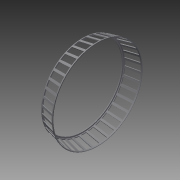
# Autodesk Inventor part: 32913_cage
Saved by Autodesk Inventor 2014 SP2 (Build 180246200, 246)
## iProperties
Created: 2018-11-17
Part Number: 32913_cage
Material: Generic
Catalog Web Link: www.cadenas.de
Description: BT1_001_101_cage-Tapered roller bearings, single row
Vendor: SKF
Document SubType Name: Modeling
Designer: psadmin
Manufacturer: SKF
Mass: 1.11318 g
Surface Area: 45.7917 cm^2
Volume: 1.11318 cm^3
Density: 1 g/cm^3
Appearance: PSOLRGB-175-175-175
Category: PARTsolutions
Company: SKF
Title: 32913_cage
Author: Cadenas PARTsolutions
Comments: Tapered roller bearings, single row
PSOL_IDENT_0: {$CADENAS_DATA\23d-libs\skf\bearings_units_and_housings\roller_bearings\tapered_roller_bearings\tape
PSOL_IDENT_1: red_roller_bearings_single_row\parts\bt1_001_101_cage.prj},172 {VTYP=3D},{NB=32913_cage},{LINA=32913
PSOL_IDENT_2: _cage},{NN=BT1_001_101_cage},{DATE=14.08.2018 07:35:10},{GEOMDATE=27.06.2018 08:15:48},{VERSION=},{L
PSOL_IDENT_3: INEID=3110},{WBVAR=},{WBNUMERIC=}  {NB=32913_cage},{LINA=32913_cage},{KT=DUMMY},{DESIGNATION=32913},
PSOL_IDENT_4: {DD=65.000},{D=90.000},{T=17.000},{DD1=78.8000},{D1=MIN},{B=17.000},{C=14.000},{C1=MIN},{R12=1.0},{R
PSOL_IDENT_5: 34=1.0},{AA=16.53733},{PITCH=77.207},{DW=5.200},{LW=12.200},{RANGLE=1.600},{ALPHA=13.250},{DDAMAX=71
PSOL_IDENT_6: },{DDAMIN=73.0},{DAMIN=83},{DAMAX=83.0},{DBMIN=86},{CA=3},{CB=3.0},{RA=1.0},{RB=1.0},{LOAD1=54.700},
PSOL_IDENT_7: {LOAD2=80.000},{LOAD3=8.150},{SPEED1=5600},{SPEED2=6700},{EE=0.35},{Y=1.70},{Y0=0.9},{Y1=0},{X1=1},{
PSOL_IDENT_8: X2=0.4},{X0=0.5},{Z=36},{II=1},{R1=0.00000231},{R2=10.9},{S1=0.009},{S2=2},{KZ=6},{KL=0.7},{BF=2},{M
PSOL_IDENT_9: ASS=0.323},{PIM=PIM_BT1_001},{DESIGN=trb1},{HELP=0.000}
NN: BT1_001_101_cage
NT: Tapered roller bearings, single row
NB: 32913_cage
NBSYN: $DESIGNATION._cage
LINA: 32913_cage
DESIGNATION: 32913
DD: 65
D: 90
T: 17
DD1: 78.8
D1: 0
B: 17
C: 14
C1: 0
R12: 1
R34: 1
AA: 16.53733
PITCH: 77.207
DW: 5.2
LW: 12.2
RANGLE: 1.6
ALPHA: 13.25
DDAMAX: 71
DDAMIN: 73
DAMIN: 83
DAMAX: 83
DBMIN: 86
CA: 3
CB: 3
RA: 1
RB: 1
LOAD1: 54.7
LOAD2: 80
LOAD3: 8.15
SPEED1: 5600
SPEED2: 6700
EE: 0.35
Y: 1.7
Y0: 0.9
Y1: 0
X1: 1
X2: 0.4
X0: 0.5
Z: 36
II: 1
R1: 0.00000231
R2: 10.9
S1: 0.009
S2: 2
KZ: 6
KL: 0.7
BF: 2
MASS: 0.323
PIM: PIM_BT1_001
SUPPLIER: SKF
ARTICLENO: 32913_cage
BOMINFO: 32913_cage
CREATOR: CADENAS GmbH
Autodesk Inventor part; units mm, degrees
ref_plane "YZ Plane" through (0, 0, 0) normal (1, 0, 0) x (0, 1, 0)
ref_plane "XZ Plane" through (0, 0, 0) normal (0, 1, 0) x (-1, 0, 0)
ref_plane "XY Plane" through (0, 0, 0) normal (0, 0, 1) x (1, 0, 0)
sketch "Sketch_1" plane through (0, 0, 0) normal (0, 0, 1) x (1, 0, 0)
  line L0 (0.4725, 0) -> (-0.1775, 0)
  line L1 (-0.1775, 38.1882) -> (-0.1775, 36.9611)
  line L2 (-0.1775, 36.9611) -> (0.4725, 36.9611)
  line L3 (0.4725, 36.9611) -> (0.4725, 38.1882)
  line L4 (0.4725, 38.1882) -> (14.3525, 41.565)
  line L5 (14.3525, 41.565) -> (14.2035, 42.1977)
  line L6 (14.2035, 42.1977) -> (0.3189, 38.8198)
  arc A0 (0.3189, 38.8198) -> (-0.1775, 38.1882) centre (0.4725, 38.1882) ccw
  constraints: 14 end point, 2 point on circle, 1 centre point
revolve "Revolution1" add sketch "Sketch_1" angle 360 about axis through (0.4725, 0, 0) along (1, 0, 0)
sketch "Sketch_2" plane through (7.1413, 0, 0) normal (1, 0, 0) x (0, 0, -1)
  line L0 (-43.8035, -2.7696) -> (-19.2633, -1.218)
  arc A0 (-19.2633, -1.218) -> (-19.1821, -2.1456) centre (0, 0) ccw
  line L1 (-19.1821, -2.1456) -> (-43.619, -4.8789)
  line L2 (-43.619, -4.8789) -> (-42.6571, -10.3339)
  line L3 (-42.6571, -10.3339) -> (-18.7591, -4.5445)
  arc A1 (-18.7591, -4.5445) -> (-18.5181, -5.4439) centre (0, 0) ccw
  line L4 (-18.5181, -5.4439) -> (-42.1091, -12.3791)
  line L5 (-42.1091, -12.3791) -> (-40.2146, -17.5842)
  line L6 (-40.2146, -17.5842) -> (-17.685, -7.7329)
  arc A2 (-17.685, -7.7329) -> (-17.2915, -8.5769) centre (0, 0) ccw
  line L7 (-17.2915, -8.5769) -> (-39.3197, -19.5032)
  line L8 (-39.3197, -19.5032) -> (-36.5502, -24.3003)
  line L9 (-36.5502, -24.3003) -> (-16.0735, -10.6864)
  arc A3 (-16.0735, -10.6864) -> (-15.5394, -11.4492) centre (0, 0) ccw
  line L10 (-15.5394, -11.4492) -> (-35.3357, -26.0347)
  line L11 (-35.3357, -26.0347) -> (-31.7752, -30.278)
  line L12 (-31.7752, -30.278) -> (-13.9736, -13.3152)
  arc A4 (-13.9736, -13.3152) -> (-13.3152, -13.9736) centre (0, 0) ccw
  line L13 (-13.3152, -13.9736) -> (-30.278, -31.7752)
  line L14 (-30.278, -31.7752) -> (-26.0347, -35.3357)
  line L15 (-26.0347, -35.3357) -> (-11.4492, -15.5394)
  arc A5 (-11.4492, -15.5394) -> (-10.6864, -16.0735) centre (0, 0) ccw
  line L16 (-10.6864, -16.0735) -> (-24.3003, -36.5502)
  line L17 (-24.3003, -36.5502) -> (-19.5032, -39.3197)
  line L18 (-19.5032, -39.3197) -> (-8.5769, -17.2915)
  arc A6 (-8.5769, -17.2915) -> (-7.7329, -17.685) centre (0, 0) ccw
  line L19 (-7.7329, -17.685) -> (-17.5842, -40.2146)
  line L20 (-17.5842, -40.2146) -> (-12.3791, -42.1091)
  line L21 (-12.3791, -42.1091) -> (-5.4439, -18.5181)
  arc A7 (-5.4439, -18.5181) -> (-4.5445, -18.7591) centre (0, 0) ccw
  line L22 (-4.5445, -18.7591) -> (-10.3339, -42.6571)
  line L23 (-10.3339, -42.6571) -> (-4.8789, -43.619)
  line L24 (-4.8789, -43.619) -> (-2.1456, -19.1821)
  arc A8 (-2.1456, -19.1821) -> (-1.218, -19.2633) centre (0, 0) ccw
  line L25 (-1.218, -19.2633) -> (-2.7696, -43.8035)
  line L26 (-2.7696, -43.8035) -> (2.7696, -43.8035)
  line L27 (2.7696, -43.8035) -> (1.218, -19.2633)
  arc A9 (1.218, -19.2633) -> (2.1456, -19.1821) centre (0, 0) ccw
  line L28 (2.1456, -19.1821) -> (4.8789, -43.619)
  line L29 (4.8789, -43.619) -> (10.3339, -42.6571)
  line L30 (10.3339, -42.6571) -> (4.5445, -18.7591)
  arc A10 (4.5445, -18.7591) -> (5.4439, -18.5181) centre (0, 0) ccw
  line L31 (5.4439, -18.5181) -> (12.3791, -42.1091)
  line L32 (12.3791, -42.1091) -> (17.5842, -40.2146)
  line L33 (17.5842, -40.2146) -> (7.7329, -17.685)
  arc A11 (7.7329, -17.685) -> (8.5769, -17.2915) centre (0, 0) ccw
  line L34 (8.5769, -17.2915) -> (19.5032, -39.3197)
  line L35 (19.5032, -39.3197) -> (24.3003, -36.5502)
  line L36 (24.3003, -36.5502) -> (10.6864, -16.0735)
  arc A12 (10.6864, -16.0735) -> (11.4492, -15.5394) centre (0, 0) ccw
  line L37 (11.4492, -15.5394) -> (26.0347, -35.3357)
  line L38 (26.0347, -35.3357) -> (30.278, -31.7752)
  line L39 (30.278, -31.7752) -> (13.3152, -13.9736)
  arc A13 (13.3152, -13.9736) -> (13.9736, -13.3152) centre (0, 0) ccw
  line L40 (13.9736, -13.3152) -> (31.7752, -30.278)
  line L41 (31.7752, -30.278) -> (35.3357, -26.0347)
  line L42 (35.3357, -26.0347) -> (15.5394, -11.4492)
  arc A14 (15.5394, -11.4492) -> (16.0735, -10.6864) centre (0, 0) ccw
  line L43 (16.0735, -10.6864) -> (36.5502, -24.3003)
  line L44 (36.5502, -24.3003) -> (39.3197, -19.5032)
  line L45 (39.3197, -19.5032) -> (17.2915, -8.5769)
  arc A15 (17.2915, -8.5769) -> (17.685, -7.7329) centre (0, 0) ccw
  line L46 (17.685, -7.7329) -> (40.2146, -17.5842)
  line L47 (40.2146, -17.5842) -> (42.1091, -12.3791)
  line L48 (42.1091, -12.3791) -> (18.5181, -5.4439)
  arc A16 (18.5181, -5.4439) -> (18.7591, -4.5445) centre (0, 0) ccw
  line L49 (18.7591, -4.5445) -> (42.6571, -10.3339)
  line L50 (42.6571, -10.3339) -> (43.619, -4.8789)
  line L51 (43.619, -4.8789) -> (19.1821, -2.1456)
  arc A17 (19.1821, -2.1456) -> (19.2633, -1.218) centre (0, 0) ccw
  line L52 (19.2633, -1.218) -> (43.8035, -2.7696)
  line L53 (43.8035, -2.7696) -> (43.8035, 2.7696)
  line L54 (43.8035, 2.7696) -> (19.2633, 1.218)
  arc A18 (19.2633, 1.218) -> (19.1821, 2.1456) centre (0, 0) ccw
  line L55 (19.1821, 2.1456) -> (43.619, 4.8789)
  line L56 (43.619, 4.8789) -> (42.6571, 10.3339)
  line L57 (42.6571, 10.3339) -> (18.7591, 4.5445)
  arc A19 (18.7591, 4.5445) -> (18.5181, 5.4439) centre (0, 0) ccw
  line L58 (18.5181, 5.4439) -> (42.1091, 12.3791)
  line L59 (42.1091, 12.3791) -> (40.2146, 17.5842)
  line L60 (40.2146, 17.5842) -> (17.685, 7.7329)
  arc A20 (17.685, 7.7329) -> (17.2915, 8.5769) centre (0, 0) ccw
  line L61 (17.2915, 8.5769) -> (39.3197, 19.5032)
  line L62 (39.3197, 19.5032) -> (36.5502, 24.3003)
  line L63 (36.5502, 24.3003) -> (16.0735, 10.6864)
  arc A21 (16.0735, 10.6864) -> (15.5394, 11.4492) centre (0, 0) ccw
  line L64 (15.5394, 11.4492) -> (35.3357, 26.0347)
  line L65 (35.3357, 26.0347) -> (31.7752, 30.278)
  line L66 (31.7752, 30.278) -> (13.9736, 13.3152)
  arc A22 (13.9736, 13.3152) -> (13.3152, 13.9736) centre (0, 0) ccw
  line L67 (13.3152, 13.9736) -> (30.278, 31.7752)
  line L68 (30.278, 31.7752) -> (26.0347, 35.3357)
  line L69 (26.0347, 35.3357) -> (11.4492, 15.5394)
  arc A23 (11.4492, 15.5394) -> (10.6864, 16.0735) centre (0, 0) ccw
  line L70 (10.6864, 16.0735) -> (24.3003, 36.5502)
  line L71 (24.3003, 36.5502) -> (19.5032, 39.3197)
  line L72 (19.5032, 39.3197) -> (8.5769, 17.2915)
  arc A24 (8.5769, 17.2915) -> (7.7329, 17.685) centre (0, 0) ccw
  line L73 (7.7329, 17.685) -> (17.5842, 40.2146)
  line L74 (17.5842, 40.2146) -> (12.3791, 42.1091)
  line L75 (12.3791, 42.1091) -> (5.4439, 18.5181)
  arc A25 (5.4439, 18.5181) -> (4.5445, 18.7591) centre (0, 0) ccw
  line L76 (4.5445, 18.7591) -> (10.3339, 42.6571)
  line L77 (10.3339, 42.6571) -> (4.8789, 43.619)
  line L78 (4.8789, 43.619) -> (2.1456, 19.1821)
  arc A26 (2.1456, 19.1821) -> (1.218, 19.2633) centre (0, 0) ccw
  line L79 (1.218, 19.2633) -> (2.7696, 43.8035)
  line L80 (2.7696, 43.8035) -> (-2.7696, 43.8035)
  line L81 (-2.7696, 43.8035) -> (-1.218, 19.2633)
  arc A27 (-1.218, 19.2633) -> (-2.1456, 19.1821) centre (0, 0) ccw
  line L82 (-2.1456, 19.1821) -> (-4.8789, 43.619)
  line L83 (-4.8789, 43.619) -> (-10.3339, 42.6571)
  line L84 (-10.3339, 42.6571) -> (-4.5445, 18.7591)
  arc A28 (-4.5445, 18.7591) -> (-5.4439, 18.5181) centre (0, 0) ccw
  line L85 (-5.4439, 18.5181) -> (-12.3791, 42.1091)
  line L86 (-12.3791, 42.1091) -> (-17.5842, 40.2146)
  line L87 (-17.5842, 40.2146) -> (-7.7329, 17.685)
  arc A29 (-7.7329, 17.685) -> (-8.5769, 17.2915) centre (0, 0) ccw
  line L88 (-8.5769, 17.2915) -> (-19.5032, 39.3197)
  line L89 (-19.5032, 39.3197) -> (-24.3003, 36.5502)
  line L90 (-24.3003, 36.5502) -> (-10.6864, 16.0735)
  arc A30 (-10.6864, 16.0735) -> (-11.4492, 15.5394) centre (0, 0) ccw
  line L91 (-11.4492, 15.5394) -> (-26.0347, 35.3357)
  line L92 (-26.0347, 35.3357) -> (-30.278, 31.7752)
  line L93 (-30.278, 31.7752) -> (-13.3152, 13.9736)
  arc A31 (-13.3152, 13.9736) -> (-13.9736, 13.3152) centre (0, 0) ccw
  line L94 (-13.9736, 13.3152) -> (-31.7752, 30.278)
  line L95 (-31.7752, 30.278) -> (-35.3357, 26.0347)
  line L96 (-35.3357, 26.0347) -> (-15.5394, 11.4492)
  arc A32 (-15.5394, 11.4492) -> (-16.0735, 10.6864) centre (0, 0) ccw
  line L97 (-16.0735, 10.6864) -> (-36.5502, 24.3003)
  line L98 (-36.5502, 24.3003) -> (-39.3197, 19.5032)
  line L99 (-39.3197, 19.5032) -> (-17.2915, 8.5769)
  arc A33 (-17.2915, 8.5769) -> (-17.685, 7.7329) centre (0, 0) ccw
  line L100 (-17.685, 7.7329) -> (-40.2146, 17.5842)
  line L101 (-40.2146, 17.5842) -> (-42.1091, 12.3791)
  line L102 (-42.1091, 12.3791) -> (-18.5181, 5.4439)
  arc A34 (-18.5181, 5.4439) -> (-18.7591, 4.5445) centre (0, 0) ccw
  line L103 (-18.7591, 4.5445) -> (-42.6571, 10.3339)
  line L104 (-42.6571, 10.3339) -> (-43.619, 4.8789)
  line L105 (-43.619, 4.8789) -> (-19.1821, 2.1456)
  arc A35 (-19.1821, 2.1456) -> (-19.2633, 1.218) centre (0, 0) ccw
  line L106 (-19.2633, 1.218) -> (-43.8035, 2.7696)
  line L107 (-43.8035, 2.7696) -> (-43.8035, -2.7696)
  constraints: 216 end point, 72 point on circle, 36 centre point
extrude "Extrusion1" cut sketch "Sketch_2" along normal mid plane 12.19
ref_plane "cage_XY" through (0, 0, 0) normal (0, 0, 1) x (1, 0, 0)
ref_plane "cage_YZ" through (0, 0, 0) normal (1, 0, 0) x (0, 1, 0)
ref_plane "cage_ZX" through (0, 0, 0) normal (0, 1, 0) x (0, 0, 1)
ref_plane "roller1_XY" through (0, 38.6035, 0) normal (1, 0, 0) x (0, 0, -1)
ref_plane "roller1_YZ" through (0, 38.6035, 0) normal (0, 0, -1) x (0, 1, 0)
ref_plane "roller1_ZX" through (0, 38.6035, 0) normal (0, 1, 0) x (1, 0, 0)
ref_plane "roller10_XY" through (0, 0, 38.6035) normal (1, 0, 0) x (0, 1, 0)
ref_plane "roller10_YZ" through (0, 0, 38.6035) normal (0, 1, 0) x (0, 0, 1)
ref_plane "roller10_ZX" through (0, 0, 38.6035) normal (0, 0, 1) x (1, 0, 0)
ref_plane "roller11_XY" through (0, -6.7034, 38.017) normal (1, 0, 0) x (0, 0.9848078, 0.1736482)
ref_plane "roller11_YZ" through (0, -6.7034, 38.017) normal (0, 0.9848078, 0.1736482) x (0, -0.1736482, 0.9848078)
ref_plane "roller11_ZX" through (0, -6.7034, 38.017) normal (0, -0.1736482, 0.9848078) x (1, 0, 0)
ref_plane "roller12_XY" through (0, -13.2032, 36.2754) normal (1, 0, 0) x (0, 0.9396926, 0.3420201)
ref_plane "roller12_YZ" through (0, -13.2032, 36.2754) normal (0, 0.9396926, 0.3420201) x (0, -0.3420201, 0.9396926)
ref_plane "roller12_ZX" through (0, -13.2032, 36.2754) normal (0, -0.3420201, 0.9396926) x (1, 0, 0)
ref_plane "roller13_XY" through (0, -19.3017, 33.4316) normal (1, 0, 0) x (0, 0.8660254, 0.5)
ref_plane "roller13_YZ" through (0, -19.3017, 33.4316) normal (0, 0.8660254, 0.5) x (0, -0.5, 0.8660254)
ref_plane "roller13_ZX" through (0, -19.3017, 33.4316) normal (0, -0.5, 0.8660254) x (1, 0, 0)
ref_plane "roller14_XY" through (0, -24.8139, 29.572) normal (1, 0, 0) x (0, 0.7660444, 0.6427876)
ref_plane "roller14_YZ" through (0, -24.8139, 29.572) normal (0, 0.7660444, 0.6427876) x (0, -0.6427876, 0.7660444)
ref_plane "roller14_ZX" through (0, -24.8139, 29.572) normal (0, -0.6427876, 0.7660444) x (1, 0, 0)
ref_plane "roller15_XY" through (0, -29.572, 24.8139) normal (1, 0, 0) x (0, 0.6427876, 0.7660444)
ref_plane "roller15_YZ" through (0, -29.572, 24.8139) normal (0, 0.6427876, 0.7660444) x (0, -0.7660444, 0.6427876)
ref_plane "roller15_ZX" through (0, -29.572, 24.8139) normal (0, -0.7660444, 0.6427876) x (1, 0, 0)
ref_plane "roller16_XY" through (0, -33.4316, 19.3017) normal (1, 0, 0) x (0, 0.5, 0.8660254)
ref_plane "roller16_YZ" through (0, -33.4316, 19.3017) normal (0, 0.5, 0.8660254) x (0, -0.8660254, 0.5)
ref_plane "roller16_ZX" through (0, -33.4316, 19.3017) normal (0, -0.8660254, 0.5) x (1, 0, 0)
ref_plane "roller17_XY" through (0, -36.2754, 13.2032) normal (1, 0, 0) x (0, 0.3420201, 0.9396926)
ref_plane "roller17_YZ" through (0, -36.2754, 13.2032) normal (0, 0.3420201, 0.9396926) x (0, -0.9396926, 0.3420201)
ref_plane "roller17_ZX" through (0, -36.2754, 13.2032) normal (0, -0.9396926, 0.3420201) x (1, 0, 0)
ref_plane "roller18_XY" through (0, -38.017, 6.7034) normal (1, 0, 0) x (0, 0.1736482, 0.9848078)
ref_plane "roller18_YZ" through (0, -38.017, 6.7034) normal (0, 0.1736482, 0.9848078) x (0, -0.9848078, 0.1736482)
ref_plane "roller18_ZX" through (0, -38.017, 6.7034) normal (0, -0.9848078, 0.1736482) x (1, 0, 0)
ref_plane "roller19_XY" through (0, -38.6035, 0) normal (1, 0, 0) x (0, 0, 1)
ref_plane "roller19_YZ" through (0, -38.6035, 0) normal (0, 0, 1) x (0, -1, 0)
ref_plane "roller19_ZX" through (0, -38.6035, 0) normal (0, -1, 0) x (1, 0, 0)
ref_plane "roller2_XY" through (0, 38.017, 6.7034) normal (1, 0, 0) x (0, 0.1736482, -0.9848078)
ref_plane "roller2_YZ" through (0, 38.017, 6.7034) normal (0, 0.1736482, -0.9848078) x (0, 0.9848078, 0.1736482)
ref_plane "roller2_ZX" through (0, 38.017, 6.7034) normal (0, 0.9848078, 0.1736482) x (1, 0, 0)
ref_plane "roller20_XY" through (0, -38.017, -6.7034) normal (1, 0, 0) x (0, -0.1736482, 0.9848078)
ref_plane "roller20_YZ" through (0, -38.017, -6.7034) normal (0, -0.1736482, 0.9848078) x (0, -0.9848078, -0.1736482)
ref_plane "roller20_ZX" through (0, -38.017, -6.7034) normal (0, -0.9848078, -0.1736482) x (1, 0, 0)
ref_plane "roller21_XY" through (0, -36.2754, -13.2032) normal (1, 0, 0) x (0, -0.3420201, 0.9396926)
ref_plane "roller21_YZ" through (0, -36.2754, -13.2032) normal (0, -0.3420201, 0.9396926) x (0, -0.9396926, -0.3420201)
ref_plane "roller21_ZX" through (0, -36.2754, -13.2032) normal (0, -0.9396926, -0.3420201) x (1, 0, 0)
ref_plane "roller22_XY" through (0, -33.4316, -19.3017) normal (1, 0, 0) x (0, -0.5, 0.8660254)
ref_plane "roller22_YZ" through (0, -33.4316, -19.3017) normal (0, -0.5, 0.8660254) x (0, -0.8660254, -0.5)
ref_plane "roller22_ZX" through (0, -33.4316, -19.3017) normal (0, -0.8660254, -0.5) x (1, 0, 0)
ref_plane "roller23_XY" through (0, -29.572, -24.8139) normal (1, 0, 0) x (0, -0.6427876, 0.7660444)
ref_plane "roller23_YZ" through (0, -29.572, -24.8139) normal (0, -0.6427876, 0.7660444) x (0, -0.7660444, -0.6427876)
ref_plane "roller23_ZX" through (0, -29.572, -24.8139) normal (0, -0.7660444, -0.6427876) x (1, 0, 0)
ref_plane "roller24_XY" through (0, -24.8139, -29.572) normal (1, 0, 0) x (0, -0.7660444, 0.6427876)
ref_plane "roller24_YZ" through (0, -24.8139, -29.572) normal (0, -0.7660444, 0.6427876) x (0, -0.6427876, -0.7660444)
ref_plane "roller24_ZX" through (0, -24.8139, -29.572) normal (0, -0.6427876, -0.7660444) x (1, 0, 0)
ref_plane "roller25_XY" through (0, -19.3017, -33.4316) normal (1, 0, 0) x (0, -0.8660254, 0.5)
ref_plane "roller25_YZ" through (0, -19.3017, -33.4316) normal (0, -0.8660254, 0.5) x (0, -0.5, -0.8660254)
ref_plane "roller25_ZX" through (0, -19.3017, -33.4316) normal (0, -0.5, -0.8660254) x (1, 0, 0)
ref_plane "roller26_XY" through (0, -13.2032, -36.2754) normal (1, 0, 0) x (0, -0.9396926, 0.3420201)
ref_plane "roller26_YZ" through (0, -13.2032, -36.2754) normal (0, -0.9396926, 0.3420201) x (0, -0.3420201, -0.9396926)
ref_plane "roller26_ZX" through (0, -13.2032, -36.2754) normal (0, -0.3420201, -0.9396926) x (1, 0, 0)
ref_plane "roller27_XY" through (0, -6.7034, -38.017) normal (1, 0, 0) x (0, -0.9848078, 0.1736482)
ref_plane "roller27_YZ" through (0, -6.7034, -38.017) normal (0, -0.9848078, 0.1736482) x (0, -0.1736482, -0.9848078)
ref_plane "roller27_ZX" through (0, -6.7034, -38.017) normal (0, -0.1736482, -0.9848078) x (1, 0, 0)
ref_plane "roller28_XY" through (0, 0, -38.6035) normal (1, 0, 0) x (0, -1, 0)
ref_plane "roller28_YZ" through (0, 0, -38.6035) normal (0, -1, 0) x (0, 0, -1)
ref_plane "roller28_ZX" through (0, 0, -38.6035) normal (0, 0, -1) x (1, 0, 0)
ref_plane "roller29_XY" through (0, 6.7034, -38.017) normal (1, 0, 0) x (0, -0.9848078, -0.1736482)
ref_plane "roller29_YZ" through (0, 6.7034, -38.017) normal (0, -0.9848078, -0.1736482) x (0, 0.1736482, -0.9848078)
ref_plane "roller29_ZX" through (0, 6.7034, -38.017) normal (0, 0.1736482, -0.9848078) x (1, 0, 0)
ref_plane "roller3_XY" through (0, 36.2754, 13.2032) normal (1, 0, 0) x (0, 0.3420201, -0.9396926)
ref_plane "roller3_YZ" through (0, 36.2754, 13.2032) normal (0, 0.3420201, -0.9396926) x (0, 0.9396926, 0.3420201)
ref_plane "roller3_ZX" through (0, 36.2754, 13.2032) normal (0, 0.9396926, 0.3420201) x (1, 0, 0)
ref_plane "roller30_XY" through (0, 13.2032, -36.2754) normal (1, 0, 0) x (0, -0.9396926, -0.3420201)
ref_plane "roller30_YZ" through (0, 13.2032, -36.2754) normal (0, -0.9396926, -0.3420201) x (0, 0.3420201, -0.9396926)
ref_plane "roller30_ZX" through (0, 13.2032, -36.2754) normal (0, 0.3420201, -0.9396926) x (1, 0, 0)
ref_plane "roller31_XY" through (0, 19.3017, -33.4316) normal (1, 0, 0) x (0, -0.8660254, -0.5)
ref_plane "roller31_YZ" through (0, 19.3017, -33.4316) normal (0, -0.8660254, -0.5) x (0, 0.5, -0.8660254)
ref_plane "roller31_ZX" through (0, 19.3017, -33.4316) normal (0, 0.5, -0.8660254) x (1, 0, 0)
ref_plane "roller32_XY" through (0, 24.8139, -29.572) normal (1, 0, 0) x (0, -0.7660444, -0.6427876)
ref_plane "roller32_YZ" through (0, 24.8139, -29.572) normal (0, -0.7660444, -0.6427876) x (0, 0.6427876, -0.7660444)
ref_plane "roller32_ZX" through (0, 24.8139, -29.572) normal (0, 0.6427876, -0.7660444) x (1, 0, 0)
ref_plane "roller33_XY" through (0, 29.572, -24.8139) normal (1, 0, 0) x (0, -0.6427876, -0.7660444)
ref_plane "roller33_YZ" through (0, 29.572, -24.8139) normal (0, -0.6427876, -0.7660444) x (0, 0.7660444, -0.6427876)
ref_plane "roller33_ZX" through (0, 29.572, -24.8139) normal (0, 0.7660444, -0.6427876) x (1, 0, 0)
ref_plane "roller34_XY" through (0, 33.4316, -19.3017) normal (1, 0, 0) x (0, -0.5, -0.8660254)
ref_plane "roller34_YZ" through (0, 33.4316, -19.3017) normal (0, -0.5, -0.8660254) x (0, 0.8660254, -0.5)
ref_plane "roller34_ZX" through (0, 33.4316, -19.3017) normal (0, 0.8660254, -0.5) x (1, 0, 0)
ref_plane "roller35_XY" through (0, 36.2754, -13.2032) normal (1, 0, 0) x (0, -0.3420201, -0.9396926)
ref_plane "roller35_YZ" through (0, 36.2754, -13.2032) normal (0, -0.3420201, -0.9396926) x (0, 0.9396926, -0.3420201)
ref_plane "roller35_ZX" through (0, 36.2754, -13.2032) normal (0, 0.9396926, -0.3420201) x (1, 0, 0)
ref_plane "roller36_XY" through (0, 38.017, -6.7034) normal (1, 0, 0) x (0, -0.1736482, -0.9848078)
ref_plane "roller36_YZ" through (0, 38.017, -6.7034) normal (0, -0.1736482, -0.9848078) x (0, 0.9848078, -0.1736482)
ref_plane "roller36_ZX" through (0, 38.017, -6.7034) normal (0, 0.9848078, -0.1736482) x (1, 0, 0)
ref_plane "roller4_XY" through (0, 33.4316, 19.3017) normal (1, 0, 0) x (0, 0.5, -0.8660254)
ref_plane "roller4_YZ" through (0, 33.4316, 19.3017) normal (0, 0.5, -0.8660254) x (0, 0.8660254, 0.5)
ref_plane "roller4_ZX" through (0, 33.4316, 19.3017) normal (0, 0.8660254, 0.5) x (1, 0, 0)
ref_plane "roller5_XY" through (0, 29.572, 24.8139) normal (1, 0, 0) x (0, 0.6427876, -0.7660444)
ref_plane "roller5_YZ" through (0, 29.572, 24.8139) normal (0, 0.6427876, -0.7660444) x (0, 0.7660444, 0.6427876)
ref_plane "roller5_ZX" through (0, 29.572, 24.8139) normal (0, 0.7660444, 0.6427876) x (1, 0, 0)
ref_plane "roller6_XY" through (0, 24.8139, 29.572) normal (1, 0, 0) x (0, 0.7660444, -0.6427876)
ref_plane "roller6_YZ" through (0, 24.8139, 29.572) normal (0, 0.7660444, -0.6427876) x (0, 0.6427876, 0.7660444)
ref_plane "roller6_ZX" through (0, 24.8139, 29.572) normal (0, 0.6427876, 0.7660444) x (1, 0, 0)
ref_plane "roller7_XY" through (0, 19.3017, 33.4316) normal (1, 0, 0) x (0, 0.8660254, -0.5)
ref_plane "roller7_YZ" through (0, 19.3017, 33.4316) normal (0, 0.8660254, -0.5) x (0, 0.5, 0.8660254)
ref_plane "roller7_ZX" through (0, 19.3017, 33.4316) normal (0, 0.5, 0.8660254) x (1, 0, 0)
ref_plane "roller8_XY" through (0, 13.2032, 36.2754) normal (1, 0, 0) x (0, 0.9396926, -0.3420201)
ref_plane "roller8_YZ" through (0, 13.2032, 36.2754) normal (0, 0.9396926, -0.3420201) x (0, 0.3420201, 0.9396926)
ref_plane "roller8_ZX" through (0, 13.2032, 36.2754) normal (0, 0.3420201, 0.9396926) x (1, 0, 0)
ref_plane "roller9_XY" through (0, 6.7034, 38.017) normal (1, 0, 0) x (0, 0.9848078, -0.1736482)
ref_plane "roller9_YZ" through (0, 6.7034, 38.017) normal (0, 0.9848078, -0.1736482) x (0, 0.1736482, 0.9848078)
ref_plane "roller9_ZX" through (0, 6.7034, 38.017) normal (0, 0.1736482, 0.9848078) x (1, 0, 0)
body "Solid1"
